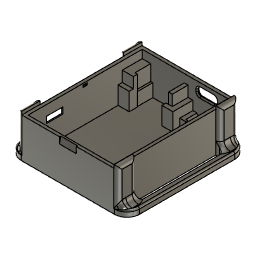
case 5.3 v6 (Autodesk Fusion 360 design; units mm, degrees)
Autodesk Fusion 360 part; units mm, degrees
note: some values were not read from the file. Set by a fixed rule: which face or edge a step refers to.
sketch "case" plane through (0, 0, 0) normal (0, 0, 1) x (1, 0, 0) in component "case"
  line L0 (0, 0) -> (41, 0)
  line L1 (41, 0) -> (41, 41)
  line L2 (0, 41) -> (0, 0)
  line L3 (0, 41) -> (0, 54.6)
  line L4 (0, 54.6) -> (41, 54.6)
  line L5 (41, 54.6) -> (41, 41)
  line L6 (4.1, 47.05) -> (0, 47.05)
  line L7 (4.1, 47.05) -> (4.1, 54.6)
  line L8 (20.15, 47.05) -> (4.1, 47.05)
  line L9 (20.15, 54.6) -> (20.15, 47.05)
  line L10 (0, 45.05) -> (5.3, 45.05)
  line L11 (5.3, 45.05) -> (5.3, 47.05)
  line L12 (12.125, 47.05) -> (12.125, 54.6) construction
  line L13 (24.25, 45.05) -> (18.95, 45.05)
  line L14 (18.95, 45.05) -> (18.95, 47.05)
  line L15 (20.15, 47.05) -> (24.25, 47.05)
  line L16 (24.25, 45.05) -> (24.25, 54.6)
  line L17 (41, 41) -> (0.0428, 41) construction
  line L18 (39, 43) -> (39, 54.6)
  line L19 (41, 41) -> (36, 41)
  line L20 (36, 41) -> (36, 43)
  line L21 (36, 43) -> (39, 43)
  line L22 (5.1, 47.05) -> (5.1, 54.6)
  line L23 (19.15, 47.05) -> (19.15, 54.6)
  line L24 (36, 43) -> (36, 45)
  line L25 (36, 45) -> (39, 45)
  line L26 (39, 43) -> (41, 43)
  line L27 (0, 2) -> (41, 2)
  line L28 (0, 43.05) -> (5.3, 43.05)
  line L29 (5.3, 45.05) -> (5.3, 43.05)
  dimension "d1" = 41
  dimension "d2" = 41
  dimension "d268" = 16.05
  dimension "d269" = 7.55
  dimension "d270" = 13.6
  dimension "d274" = 2
  dimension "d275" = 1.2
  dimension "d329" = 2
  dimension "d330" = 2
  dimension "d336" = 4.1
  dimension "d338" = 1
  dimension "d373" = 2
  dimension "d374" = 5
  dimension "d375" = 2
  dimension "d494" = 2
  constraint horizontal L0
  constraint vertical L1
  constraint vertical L2
  constraint coincident L0.start L2.end
  constraint vertical L3
  constraint horizontal L4
  constraint vertical L5
  constraint vertical L9
  constraint horizontal L8
  constraint vertical L7
  constraint perpendicular L6 L7
  constraint coincident L3 L6.end
  constraint coincident L4 L7.end
  constraint coincident L4 L9.start
  constraint coincident L3 L10.start
  constraint perpendicular L3 L10
  constraint coincident L8 L11.end
  constraint perpendicular L8 L11
  constraint midpoint L8 L12.start
  constraint coincident L4 L12.end
  constraint perpendicular L4 L12
  constraint symmetric L6.start L12 L8.start
  constraint symmetric L6.end L12 L15.end
  constraint symmetric L10.start L12 L13.start
  constraint symmetric L10.end L12 L13.end
  constraint symmetric L11.end L12 L14.end
  constraint coincident L4 L16.end
  constraint perpendicular L4 L16
  constraint perpendicular L5 L17
  constraint collinear L1.end L2.start L17.end
  constraint coincident L4 L18.end
  constraint perpendicular L4 L18
  constraint coincident L17 L19.end
  constraint perpendicular L17 L20
  constraint perpendicular L20 L21
  constraint coincident L18.start L21
  constraint coincident L8 L22.start
  constraint coincident L4 L22.end
  constraint perpendicular L4 L22
  constraint symmetric L12 L22.start L23.start
  constraint symmetric L12 L22.end L23.end
  constraint perpendicular L21 L24
  constraint coincident L18 L25.end
  constraint perpendicular L18 L25
  constraint coincident L5 L26.end
  constraint parallel L21 L26
  constraint coincident L2 L27.start
  constraint coincident L1 L27.end
  constraint perpendicular L1 L27
  constraint coincident L3 L28.start
  constraint perpendicular L3 L28
  constraint perpendicular L28 L29
  measures "d1" distance of L0.start L0.end
  measures "d2" distance of L0.start L2.start
  measures "d268" distance of L7.end L9.start
  measures "d269" distance of L6.start L7.end
  measures "d270" distance of L2.start L4
  measures "d274" distance of L6 L10
  measures "d275" distance of L7 L11
  measures "d329" distance of L5 L18
  measures "d330" distance of L19 L21
  measures "d336" distance of L3 L7
  measures "d338" distance of L7 L22
  measures "d373" distance of L21 L25
  measures "d374" distance of L5 L24
  measures "d375" distance of L0 L27
  measures "d494" distance of L10 L28
extrude "Extrude1" add sketch "case" along normal blind 17.5 makes body 1 in component "case"
shell "Shell1" thickness 1.5 outward yes removed faces 1 at (13.6667, 28, 17.5) on bodies 1 in component "case"
extrude "Extrude21" add sketch "case" along normal blind 8.5 contours L0 L1 L2 L27 | L3 L10 L28 L29 | L4 L5 L18 L26 | L18 L21 L24 L25 | L4 L9 L15 L16 | L8 L13 L14 L15 L16 bodies 1 in component "case"
extrude "Extrude22" add sketch "case" along normal blind 13.6 contours L3 L6 L8 L10 L11 | L3 L4 L6 L7 bodies 1 in component "case"
extrude "Extrude25" add sketch "case" along normal blind 6.2 contours L4 L7 L8 L22 | L4 L8 L9 L23 bodies 1 in component "case"
sketch "tray" plane through (0, 0, 0) normal (0, 0, 1) x (1, 0, 0) in component "tray"
  line L0 (0, 0) -> (40.75, 0)
  line L1 (40.75, 0) -> (40.75, 54.3)
  line L2 (0, 54.3) -> (0, 0)
  line L3 (25.45, 25.8) -> (25.45, 27.6)
  line L4 (25.45, 27.6) -> (36.25, 27.6)
  line L5 (36.25, 27.6) -> (36.25, 25.8)
  line L6 (36.25, 25.8) -> (25.45, 27.6) construction
  line L7 (25.45, 25.8) -> (36.25, 27.6) construction
  line L8 (0, 43.7) -> (0, 27.5) construction
  line L9 (0, 54.3) -> (0, 43.7)
  line L10 (40.75, 54.3) -> (0, 54.3)
  line L11 (0, 25.8) -> (40.75, 25.8)
  line L12 (0, 12.9) -> (40.75, 12.9) construction
  line L13 (27.2, 6.65) -> (11.5, 6.65)
  line L14 (11.5, 6.65) -> (11.5, 19.15)
  line L15 (11.5, 19.15) -> (27.2, 19.15)
  line L16 (27.2, 19.15) -> (27.2, 6.65)
  line L17 (27.2, 6.65) -> (11.5, 19.15) construction
  line L18 (11.5, 6.65) -> (27.2, 19.15) construction
  line L19 (34.5, 4.7) -> (10, 4.7)
  line L20 (10, 4.7) -> (10, 21.1)
  line L21 (10, 21.1) -> (34.5, 21.1)
  line L22 (34.5, 21.1) -> (34.5, 4.7)
  line L23 (34.5, 4.7) -> (10, 21.1) construction
  line L24 (10, 4.7) -> (34.5, 21.1) construction
  line L25 (32.3, 25.8) -> (34.5, 23.6)
  line L26 (34.5, 21.1) -> (34.5, 25.8)
  line L27 (32.3, 0) -> (34.5, 2.2)
  line L28 (34.5, 4.7) -> (34.5, 0)
  line L29 (7.097, 0) -> (7.097, 3)
  line L30 (7.097, 3) -> (28.483, 3)
  line L31 (28.483, 3) -> (28.483, 0)
  line L32 (7.097, 0) -> (28.483, 0)
  line L33 (7.097, 25.8) -> (28.483, 25.8)
  line L34 (28.483, 22.8) -> (28.483, 25.8)
  line L35 (7.097, 22.8) -> (28.483, 22.8)
  line L36 (7.097, 25.8) -> (7.097, 22.8)
  line L37 (39.55, 25.8) -> (39.55, 54.3)
  line L38 (39.55, 40.05) -> (22.15, 40.05) construction
  line L39 (22.15, 25.8) -> (22.15, 54.3)
  line L40 (30.85, 40.05) -> (30.85, 25.8) construction
  line L41 (34.5, 23.6) -> (40.75, 23.6)
  line L42 (36.15, 54.3) -> (36.15, 50.9)
  line L43 (36.15, 50.9) -> (39.55, 50.9)
  line L44 (25.55, 50.9) -> (22.15, 50.9)
  line L45 (25.55, 54.3) -> (25.55, 50.9)
  line L46 (22.15, 27.9) -> (39.55, 27.9)
  line L47 (22.15, 31.3) -> (39.55, 31.3)
  line L48 (0, 25.8) -> (0, 0) construction
  line L49 (25.45, 25.8) -> (36.25, 25.8)
  line L50 (4.2, 54.3) -> (20.2, 54.3)
  line L51 (20.2, 54.3) -> (20.2, 46.5)
  line L52 (20.2, 46.5) -> (4.2, 46.5)
  line L53 (4.2, 46.5) -> (4.2, 54.3)
  line L54 (4.2, 46.5) -> (0, 46.5)
  line L55 (20.2, 46.5) -> (22.15, 46.5)
  line L56 (20.8, 46.5) -> (20.8, 25.8)
  line L57 (0, 42.9) -> (20.8, 42.9)
  line L58 (0, 27) -> (20.8, 27)
  line L59 (20.8, 39.9) -> (10, 39.9)
  line L60 (10, 39.9) -> (10, 42.9)
  line L61 (20.8, 46.5) -> (20.8, 54.3)
  line L62 (22.15, 50.9) -> (20.8, 50.9)
  line L63 (0, 44.1) -> (5.2, 44.1)
  line L64 (5.2, 44.1) -> (5.2, 42.9)
  line L65 (20.8, 27) -> (22.15, 27)
  line L66 (25.45, 27) -> (36.25, 27)
  line L67 (5.2, 44.1) -> (10, 44.1)
  line L68 (10, 42.9) -> (10, 44.1)
  circle A0 centre (18.1, 29.6) radius 1.4
  line L69 (0, 29.6) -> (20.8, 29.6) construction
  line L70 (10.4, 29.6) -> (10.4, 27)
  line L71 (20.8, 44.1) -> (18.8, 44.1)
  line L72 (18.8, 44.1) -> (18.8, 42.9)
  circle A1 centre (2.7, 29.6) radius 1.4
  line L73 (36.25, 25.8) -> (36.25, 23.6)
  line L74 (27.2, 19.15) -> (30.4, 19.15)
  line L75 (30.4, 19.15) -> (30.4, 6.65)
  line L76 (30.4, 6.65) -> (27.2, 6.65)
  line L77 (28.483, 3) -> (28.483, 22.8)
  point P0 (30.85, 26.7)
  point P1 (19.35, 12.9)
  point P2 (22.25, 12.9)
  point P3 (61.6964, 12.9)
  point P4 (8.897, 1.47)
  point P5 (26.683, 1.47)
  dimension "d38" = 40.75
  dimension "d46" = 10.8
  dimension "d141" = 12.5
  dimension "d142" = 11.5
  dimension "d143" = 27.2
  dimension "d144" = 10
  dimension "d145" = 34.5
  dimension "d146" = 16.4
  dimension "d199" = 54.3
  dimension "d212" = 8.897
  dimension "d213" = 17.786
  dimension "d214" = 1.47
  dimension "d215" = 1.8
  dimension "d216" = 1.8
  dimension "d217" = 3
  dimension "d218" = 1.47
  dimension "d222" = 17.4
  dimension "d224" = 25.8
  dimension "d226" = 3.4
  dimension "d227" = 3.4
  dimension "d229" = 23
  dimension "d244" = 26.4
  dimension "d246" = 26.7
  dimension "d247" = 45
  dimension "d248" = 1.8
  dimension "d249" = 32.3
  dimension "d253" = 1.2
  dimension "d254" = 16
  dimension "d255" = 7.8
  dimension "d256" = 4.2
  dimension "d257" = 9.9
  dimension "d259" = 20.8
  dimension "d261" = 1.2
  dimension "d262" = 15.9
  dimension "d263" = 10.8
  dimension "d264" = 3
  dimension "d265" = 5.2
  dimension "d266" = 1.2
  dimension "d323" = 2.8
  dimension "d326" = 2.6
  dimension "d353" = 2.7
  dimension "d354" = 2
  dimension "d363" = 28.5
  dimension "d364" = 2.2
  dimension "d365" = 24.5
  dimension "d366" = 1.5
  dimension "d367" = 15.7
  dimension "d459" = 3.2
  constraint horizontal L0
  constraint vertical L1
  constraint horizontal L10
  constraint collinear L0.start L2.end L0.end
  constraint coincident L6 P0
  constraint coincident L7 P0
  constraint coincident L2 L8.end
  constraint vertical L9
  constraint coincident L2 L12.start
  constraint coincident L1 L12.end
  constraint perpendicular L1 L12
  constraint horizontal L13
  constraint perpendicular L13 L14
  constraint parallel L13 L15
  constraint parallel L14 L16
  constraint coincident L17 P1
  constraint coincident L18 P1
  constraint coincident L12 P1
  constraint horizontal L19
  constraint perpendicular L19 L20
  constraint parallel L19 L21
  constraint parallel L20 L22
  constraint coincident L23 P2
  constraint coincident L24 P2
  constraint coincident L12 P2
  constraint perpendicular L21 L26
  constraint coincident L25.end L26
  constraint symmetric L12 L21.end L19.start
  constraint symmetric L12 L25.start L27.start
  constraint symmetric L12 L25.end L27.end
  constraint symmetric L12 L26.end L28.end
  constraint coincident L12 P3
  constraint coincident L0 L29.start
  constraint perpendicular L0 L29
  constraint perpendicular L29 L30
  constraint coincident L0 L31.end
  constraint perpendicular L0 L31
  constraint symmetric L12 L29.start L33.start
  constraint symmetric L12 L29.end L35.start
  constraint symmetric L12 L30.end L34.start
  constraint symmetric L12 L31.end L33.end
  constraint coincident L10 L37.end
  constraint perpendicular L10 L37
  constraint coincident L2.start L10
  constraint midpoint L37 L38.start
  constraint perpendicular L37 L38
  constraint coincident L11 L39.start
  constraint coincident L10 L39.end
  constraint perpendicular L10 L39
  constraint coincident L38.end L39
  constraint vertical L40
  constraint midpoint L38 L40.start
  constraint coincident P0 L40
  constraint coincident L1 L41.end
  constraint perpendicular L1 L41
  constraint coincident L10 L42.start
  constraint perpendicular L10 L42
  constraint coincident L37 L43.end
  constraint perpendicular L37 L43
  constraint symmetric L40 L42.start L45.start
  constraint symmetric L40 L42.end L44.start
  constraint symmetric L40 L43.end L44.end
  constraint coincident L39 L46.start
  constraint coincident L37 L46.end
  constraint perpendicular L37 L46
  constraint coincident L39 L47.start
  constraint coincident L37 L47.end
  constraint perpendicular L39 L47
  constraint midpoint L12.start L48
  constraint coincident L1 L11.end
  constraint midpoint L7 P0
  constraint perpendicular L5 L49
  constraint coincident L11 L25.start
  constraint horizontal L50
  constraint vertical L51
  constraint horizontal L52
  constraint vertical L53
  constraint coincident L10 L50.start
  constraint coincident L9 L54.end
  constraint perpendicular L53 L54
  constraint coincident L39 L55.end
  constraint perpendicular L39 L55
  constraint vertical L56
  constraint coincident L55 L56.start
  constraint coincident L11 L56.end
  constraint coincident L8 L57.start
  constraint coincident L56 L57.end
  constraint perpendicular L56 L57
  constraint coincident L2 L58.start
  constraint coincident L56 L58.end
  constraint perpendicular L56 L58
  constraint coincident L56 L59.start
  constraint perpendicular L56 L59
  constraint coincident L57 L60.end
  constraint perpendicular L57 L60
  constraint coincident L10 L61.end
  constraint perpendicular L10 L61
  constraint coincident L61 L62.end
  constraint perpendicular L61 L62
  constraint coincident L9 L63.start
  constraint perpendicular L9 L63
  constraint coincident L57 L64.end
  constraint perpendicular L57 L64
  constraint collinear L11 L49
  constraint coincident L39 L65.end
  constraint perpendicular L39 L65
  constraint coincident L3 L66.start
  constraint coincident L5 L66.end
  constraint perpendicular L5 L66
  constraint collinear L65 L66
  constraint perpendicular L56 L67
  constraint perpendicular L57 L68
  constraint coincident L67.end L68
  constraint coincident L8 L69.start
  constraint coincident L56 L69.end
  constraint perpendicular L56 L69
  constraint coincident A0.centre L69
  constraint midpoint L69 L70.start
  constraint midpoint L58 L70.end
  constraint coincident L56 L71.start
  constraint perpendicular L56 L71
  constraint coincident L57 L72.end
  constraint perpendicular L57 L72
  constraint collinear L67 L71
  constraint symmetric A0 L70 A1
  constraint coincident L41 L73.end
  constraint perpendicular L41 L73
  constraint perpendicular L16 L74
  constraint perpendicular L74 L75
  constraint perpendicular L16 L76
  constraint coincident L0.start L2.end
  measures "d38" distance of L0.start L0.end
  measures "d46" distance of L3 L5
  measures "d141" distance of L13.end L14.end
  measures "d142" distance of L2 L14
  measures "d143" distance of L2 L16
  measures "d144" distance of L2 L20
  measures "d145" distance of L2 L22
  measures "d146" distance of L19 L21
  measures "d199" distance of L0 L10
  measures "d212" distance of L2 P4
  measures "d213" distance of P4 P5
  measures "d214" distance of L0 P4
  measures "d215" distance of P4 L29
  measures "d216" distance of P5 L31
  measures "d217" distance of L0 L30
  measures "d218" distance of L0 P5
  measures "d222" distance of L38.start L38.end
  measures "d224" distance of L0 L11
  measures "d226" distance of L42.end L43.end
  measures "d227" distance of L42.start L42.end
  measures "d229" distance of L10 L47
  measures "d244" distance of L10 L46
  measures "d246" distance of L4 L10
  measures "d247" angle of L11 L25
  measures "d248" distance of L4 L11
  measures "d249" distance of L2 L25.start
  measures "d253" distance of L1 L37
  measures "d254" distance of L50.start L50.end
  measures "d255" distance of L50.start L52.end
  measures "d256" distance of L2 L53
  measures "d257" distance of L1 L40
  measures "d259" distance of L2 L56
  measures "d261" distance of L11 L58
  measures "d262" distance of L57 L58
  measures "d263" distance of L59.start L59.end
  measures "d264" distance of L59.end L60.end
  measures "d265" distance of L63.start L63.end
  measures "d266" distance of L63.end L64.end
  measures "d323" diameter of A0
  measures "d326" distance of L58 L69
  measures "d353" distance of L56 A0.centre
  measures "d354" distance of L56 L72
  measures "d363" distance of L10 L33
  measures "d364" distance of L25.end L26.end
  measures "d365" distance of L20 L22
  measures "d366" distance of L14 L20
  measures "d367" distance of L14 L16
  measures "d459" distance of L15.end L74.end
extrude "Extrude6" add sketch "tray" against normal blind 1.55 separate body contours L0 L2 L11 L19 L20 L21 L29 L30 L35 L36 L77 | L2 L11 L33 L56 L58 | L0 L19 L27 L28 L31 L77 | L2 L56 L57 L58 L59 L60 | L0 L27 L28 | L2 L9 L57 L63 L64 | L11 L33 L39 L56 L65 | L19 L21 L22 L74 L75 L76 L77 | L13 L14 L15 L19 L20 L21 L74 L76 L77 | L39 L55 L56 L65 | L3 L4 L5 L11 L33 L37 L39 L46 | L11 L21 L25 L26 L34 L49 L77 | L74 L75 L76 L77 | L16 L74 L76 L77 | L3 L5 L11 L33 L49 L66 | L1 L11 L41 L73 | L13 L14 L15 L16 | L56 L57 L71 L72 | L3 L4 L5 L66 | L11 L25 L26 L49 | L1 L10 L11 L37 | L11 L26 L41 L49 L73 | L10 L37 L39 L42 L43 L44 L45 L47 | A0 | A1 makes body 2 in component "tray"
extrude "Extrude7" add sketch "tray" along normal blind 2.4 contours L2 L9 L57 L63 L64 | L39 L55 L56 L65 | L1 L11 L41 L73 | L56 L57 L71 L72 | L3 L4 L5 L66 | L1 L10 L11 L37 | L11 L26 L41 L49 L73 bodies 2 in component "tray"
extrude "Extrude1'" add sketch "tray" along normal blind 4 contours L2 L11 L33 L56 L58 | L0 L27 L28 | L11 L33 L39 L56 L65 | L3 L5 L11 L33 L49 L66 | L11 L25 L26 L49 | L11 L26 L41 L49 L73 bodies 2 in component "tray"
extrude "Extrude15" cut sketch "tray" along normal through all from surface at -0.55 contours L0 L2 L11 L19 L20 L21 L29 L30 L35 L36 L77 | L0 L19 L27 L28 L31 L77 | L19 L21 L22 L74 L75 L76 L77 | L13 L14 L15 L19 L20 L21 L74 L76 L77 | L11 L21 L25 L26 L34 L49 L77 | L74 L75 L76 L77 | L16 L74 L76 L77 | L13 L14 L15 L16 bodies 2 in component "tray"
sketch "switch shoulder" plane through (0, 0, 8.5) normal (0, 0, 1) x (-1, 0, 0) in component "case"
  line L0 (-18.95, -45.05) -> (-24.25, -45.05)
  line L1 (-24.25, -45.05) -> (-24.25, -54.6)
  line L2 (-24.25, -54.6) -> (-20.15, -54.6)
  line L3 (-20.15, -54.6) -> (-20.15, -47.05)
  line L4 (-20.15, -47.05) -> (-18.95, -47.05)
  line L5 (-18.95, -47.05) -> (-18.95, -45.05)
  line L6 (-22.25, -51.05) -> (-25.65, -51.05)
  line L7 (-22.25, -46.65) -> (-22.25, -51.05)
  line L8 (-20.9, -46.65) -> (-22.25, -46.65)
  line L9 (-20.15, -47.05) -> (-21.95, -47.05)
  line L10 (-21.95, -47.05) -> (-21.95, -54.6)
  line L11 (-20.9, -44.25) -> (-20.9, -46.65)
  line L12 (-20.9, -40.05) -> (-20.9, -43.05)
  dimension "d304" = 1.8
  constraint coincident L3.end L4.start
  constraint perpendicular L3 L9
  constraint coincident L2 L10.end
  constraint perpendicular L2 L10
  measures "d304" distance of L3 L10
extrude "Extrude24" add sketch "switch shoulder" along normal up to surface (5.1 mm away) contours L2 L3 L9 L10 bodies 1 in component "case"
sketch "usb c" plane through (0, 54.6, 0) normal (0, -1, 0) x (1, 0, 0) in component "case"
  line L0 (0, 13.6) -> (4.1, 13.6)
  line L1 (4.1, 13.6) -> (4.1, 6.2)
  line L2 (5.1, 0) -> (19.15, 0)
  line L3 (20.15, 6.2) -> (20.15, 13.6)
  line L4 (21.95, 8.5) -> (24.25, 8.5)
  line L5 (24.25, 8.5) -> (24.25, 0)
  line L6 (24.25, 0) -> (39, 0)
  line L7 (41, 8.5) -> (41, 17.5)
  line L8 (41, 17.5) -> (0, 17.5)
  line L9 (0, 17.5) -> (0, 13.6)
  line L10 (34.2, 11.6) -> (27.6, 11.6)
  arc A0 (26.3, 12.9) -> (27.6, 11.6) centre (27.6, 12.9) ccw
  line L11 (26.3, 12.9) -> (26.3, 13.9)
  arc A1 (27.6, 15.2) -> (26.3, 13.9) centre (27.6, 13.9) ccw
  line L12 (27.6, 15.2) -> (34.2, 15.2)
  arc A2 (35.5, 13.9) -> (34.2, 15.2) centre (34.2, 13.9) ccw
  line L13 (35.5, 13.9) -> (35.5, 12.9)
  arc A3 (34.2, 11.6) -> (35.5, 12.9) centre (34.2, 12.9) ccw
  line L14 (26.3, 13.4) -> (35.5, 13.4) construction
  line L15 (24.25, 8.5) -> (41, 8.5) construction
  line L16 (30.9, 13.4) -> (30.9, 8.5) construction
  line L17 (39, 0) -> (39, 8.5)
  line L18 (39, 8.5) -> (41, 8.5)
  line L19 (5.1, 6.2) -> (5.1, 0)
  line L20 (19.15, 0) -> (19.15, 6.2)
  line L21 (19.15, 6.2) -> (20.15, 6.2)
  line L22 (4.1, 6.2) -> (5.1, 6.2)
  line L23 (30.9, 8.5) -> (30.9, 0) construction
  line L24 (21.95, 13.6) -> (21.95, 8.5)
  line L25 (20.15, 13.6) -> (21.95, 13.6)
  point P0 (30.9, 13.4)
  point P1 (30.9, 10.1)
  dimension "d280" = 9.2
  dimension "d281" = 3.6
  dimension "d282" = 1.3
  dimension "d283" = 10.1
  dimension "d288" = 1.6
  dimension "d289" = 1.5
  constraint horizontal L10
  constraint vertical L11
  constraint horizontal L12
  constraint vertical L13
  constraint tangent L12 A2
  constraint tangent A2 L13
  constraint tangent L13 A3
  constraint tangent L10 A3
  constraint equal A2 A3
  constraint tangent L10 A0
  constraint tangent A0 L11
  constraint equal A0 A2
  constraint tangent L11 A1
  constraint tangent A1 L12
  constraint equal A1 A2
  constraint midpoint L14.start L11
  constraint midpoint L14.end L13
  constraint midpoint L14 P0
  constraint coincident L4.end L5.start
  constraint coincident L7 L15.end
  constraint perpendicular L7 L15
  constraint coincident P0 L16.start
  constraint coincident L15 L16.end
  constraint perpendicular L15 L16
  constraint coincident L16 P1
  constraint coincident L6 L23.end
  constraint perpendicular L6 L23
  measures "d280" distance of L11 L13
  measures "d281" distance of L10 L12
  measures "d282" radius of A2
  measures "d283" distance of L7 P0
  measures "d288" distance of L15 P1
  measures "d289" distance of L10 P1
extrude "Extrude23" cut sketch "usb c" against normal through all contours L10 A0 L11 A1 L12 A2 L13 A3 bodies 1 in component "case"
chamfer "Chamfer3" distance 0.6 angle 45 16 edges at (30.9, 54.6, 15.2) (35.1192, 54.6, 14.8192) (35.5, 54.6, 13.4) (35.1192, 54.6, 11.9808) (30.9, 54.6, 11.6) (26.6808, 54.6, 11.9808) (26.3, 54.6, 13.4) (26.6808, 54.6, 14.8192) (30.9, 56.1, 15.2) (26.6808, 56.1, 14.8192) (26.3, 56.1, 13.4) (26.6808, 56.1, 11.9808) (30.9, 56.1, 11.6) (35.1192, 56.1, 11.9808) (35.5, 56.1, 13.4) (35.1192, 56.1, 14.8192) on bodies 1 in component "case"
sketch "lid" plane through (0, 0, 0) normal (0, 0, 1) x (1, 0, 0) in component "lid"
  line L0 (41, 54.6) -> (0, 54.6)
  line L1 (41, 54.6) -> (41, 0)
  line L2 (41, 0) -> (0, 0)
  line L3 (0, 0) -> (0, 54.6)
  line L4 (42.5, 56.1) -> (-1.5, 56.1)
  line L5 (-1.5, -1.5) -> (-1.5, 56.1)
  line L6 (42.5, -1.5) -> (-1.5, -1.5)
  line L7 (42.5, 56.1) -> (42.5, -1.5)
  line L8 (1.25, 1.25) -> (1.25, 53.35)
  line L9 (39.75, 53.35) -> (1.25, 53.35)
  line L10 (39.75, 53.35) -> (39.75, 1.25)
  line L11 (39.75, 1.25) -> (1.25, 1.25)
  line L12 (20.15, 54.6) -> (20.15, 47.05) construction
  line L13 (4.1, 47.05) -> (4.1, 54.6) construction
  line L14 (4.1, 54.6) -> (20.15, 54.6) construction
  line L15 (4.1, 47.05) -> (20.15, 47.05) construction
  line L16 (12.125, 47.05) -> (12.125, 54.6) construction
  line L17 (16.725, 48.725) -> (7.525, 48.725)
  line L18 (7.525, 48.725) -> (7.525, 52.925)
  line L19 (7.525, 52.925) -> (16.725, 52.925)
  line L20 (16.725, 52.925) -> (16.725, 48.725)
  line L21 (16.725, 48.725) -> (7.525, 52.925) construction
  line L22 (7.525, 48.725) -> (16.725, 52.925) construction
  line L23 (0, 49.35) -> (1.25, 49.35)
  line L24 (20.5, 1.25) -> (20.5, 53.35) construction
  line L25 (1.25, 27.3) -> (39.75, 27.3) construction
  line L26 (0, 33.3) -> (1.25, 33.3)
  line L27 (0, 5.25) -> (1.25, 5.25)
  line L28 (0, 21.3) -> (1.25, 21.3)
  line L29 (41, 49.35) -> (39.75, 49.35)
  line L30 (41, 33.3) -> (39.75, 33.3)
  line L31 (41, 21.3) -> (39.75, 21.3)
  line L32 (41, 5.25) -> (39.75, 5.25)
  line L33 (0.25, 0.25) -> (0.25, 54.35)
  line L34 (40.75, 54.35) -> (0.25, 54.35)
  line L35 (40.75, 54.35) -> (40.75, 0.25)
  line L36 (40.75, 0.25) -> (0.25, 0.25)
  line L37 (37, 54.35) -> (37, 53.35)
  line L38 (24.8, 54.35) -> (24.8, 53.35)
  line L39 (6.925, 48.125) -> (17.325, 48.125)
  line L40 (6.925, 48.125) -> (6.925, 53.35)
  line L41 (17.325, 48.125) -> (17.325, 53.35)
  line L42 (6.175, 47.375) -> (6.175, 53.35)
  line L43 (6.175, 47.375) -> (18.075, 47.375)
  line L44 (18.075, 47.375) -> (18.075, 53.35)
  line L45 (1.25, 53.35) -> (0.25, 53.35)
  line L46 (39.75, 53.35) -> (40.75, 53.35)
  line L47 (39.75, 1.25) -> (40.75, 1.25)
  line L48 (1.25, 1.25) -> (0.25, 1.25)
  point P0 (12.125, 50.825)
  point P1 (35.5, 54.6)
  point P2 (26.3, 54.6)
  point P3 (12.125, 48.125)
  dimension "d310" = -1.5
  dimension "d311" = 1.25
  dimension "d318" = 9.2
  dimension "d319" = 4.2
  dimension "d332" = 4
  dimension "d333" = 6
  dimension "d362" = 0.25
  dimension "d368" = 1.5
  dimension "d369" = 1.5
  dimension "d370" = 0.6
  dimension "d371" = 0.6
  dimension "d372" = -0.75
  constraint coincident L13.end L14.start
  constraint coincident L12.start L14.end
  constraint coincident L13.start L15.start
  constraint coincident L12.end L15.end
  constraint midpoint L15 L16.start
  constraint midpoint L14 L16.end
  constraint horizontal L17
  constraint perpendicular L17 L18
  constraint parallel L17 L19
  constraint parallel L18 L20
  constraint coincident L21 P0
  constraint coincident L22 P0
  constraint midpoint L16 P0
  constraint coincident L3 L23.start
  constraint coincident L8 L23.end
  constraint perpendicular L8 L23
  constraint midpoint L11 L24.start
  constraint midpoint L9 L24.end
  constraint midpoint L8 L25.start
  constraint midpoint L10 L25.end
  constraint coincident L3 L26.start
  constraint coincident L8 L26.end
  constraint perpendicular L8 L26
  constraint symmetric L23.start L25 L27.start
  constraint symmetric L23.end L25 L27.end
  constraint symmetric L25 L26.start L28.start
  constraint symmetric L25 L26.end L28.end
  constraint symmetric L23.start L24 L29.start
  constraint symmetric L23.end L24 L29.end
  constraint symmetric L24 L26.start L30.start
  constraint symmetric L24 L26.end L30.end
  constraint symmetric L24 L27.start L32.start
  constraint symmetric L24 L27.end L32.end
  constraint symmetric L24 L28.start L31.start
  constraint symmetric L24 L28.end L31.end
  constraint coincident L34 L37.start
  constraint coincident L9 L37.end
  constraint perpendicular L9 L37
  constraint coincident L34 L38.start
  constraint coincident L9 L38.end
  constraint perpendicular L9 L38
  constraint perpendicular L16 L39
  constraint midpoint L39 P3
  constraint coincident L16 P3
  constraint coincident L9 L40.end
  constraint perpendicular L9 L40
  constraint coincident L9 L41.end
  constraint perpendicular L9 L41
  constraint coincident L33 L45.end
  constraint perpendicular L33 L45
  constraint coincident L35 L46.end
  constraint perpendicular L35 L46
  constraint coincident L35 L47.end
  constraint perpendicular L35 L47
  constraint coincident L33 L48.end
  constraint perpendicular L33 L48
  measures "d318" distance of L18.end L19.end
  measures "d319" distance of L17.end L18.end
  measures "d332" distance of L9 L23
  measures "d333" distance of L25 L26
  measures "d368" distance of P2 L38
  measures "d369" distance of P1 L37
  measures "d370" distance of L17 L39
  measures "d371" distance of L20 L41
extrude "Extrude1''" add sketch "lid" along normal blind 1.5 separate body contours L0 L1 L3 L23 L29 L33 L34 L35 | L1 L29 L30 L35 | L3 L23 L26 L33 | L1 L30 L31 L35 | L10 L29 L30 L35 | L10 L29 L35 L46 | L3 L26 L28 L33 | L8 L23 L33 L45 | L8 L23 L26 L33 | L1 L31 L32 L35 | L10 L30 L31 L35 | L8 L9 L10 L11 L42 L43 L44 | L9 L34 L35 L37 L46 | L3 L27 L28 L33 | L8 L26 L28 L33 | L9 L33 L34 L38 L45 | L1 L2 L3 L27 L32 L33 L35 L36 | L10 L31 L32 L35 | L8 L27 L28 L33 | L10 L32 L35 L47 | L9 L34 L37 L38 | L8 L27 L33 L48 | L9 L39 L40 L41 L42 L43 L44 | L11 L33 L35 L36 L47 L48 | L9 L39 L40 L41 | L4 L5 L6 L7 | L17 L18 L19 L20 makes body 3 in component "lid"
extrude "Extrude2" add sketch "lid" against normal blind 1.6 contours L9 L34 L35 L37 L46 | L9 L33 L34 L38 L45 | L9 L39 L40 L41 L42 L43 L44 | L11 L33 L35 L36 L47 L48 bodies 3 in component "lid"
extrude "Extrude4" add sketch "lid" against normal blind 2.4 contours L1 L30 L31 L35 | L3 L26 L28 L33 | L10 L30 L31 L35 | L8 L26 L28 L33 bodies 3 in component "lid"
extrude "Extrude3" cut sketch "lid" along normal through all contours L17 L18 L19 L20 bodies 3 in component "lid"
chamfer "Chamfer1" distance 1 distance2 1 4 edges at (7.525, 50.825, 1.5) (12.125, 52.925, 1.5) (12.125, 48.725, 1.5) (16.725, 50.825, 1.5) measured on face at (19.2417, 15.2417, 1.5) measured on face at (19.2417, 15.2417, 1.5) measured on face at (19.2417, 15.2417, 1.5) measured on face at (19.2417, 15.2417, 1.5) on bodies 3 in component "lid"
sketch "snap pins" plane through (0, 0, -17) normal (-1, 0, 0) x (0, -1, 0) in component "lid"
  line L0 (-21.3, 17) -> (-33.3, 17)
  line L1 (-33.3, 17) -> (-33.3, 14.6)
  line L2 (-33.3, 14.6) -> (-21.3, 14.6)
  line L3 (-21.3, 14.6) -> (-21.3, 17)
  line L4 (-33.3, 15.8) -> (-21.3, 15.8) construction
  line L5 (-26.5, 15.5) -> (-28.1, 15.5)
  line L6 (-28.1, 15.5) -> (-28.1, 16.1)
  line L7 (-28.1, 16.1) -> (-26.5, 16.1)
  line L8 (-26.5, 16.1) -> (-26.5, 15.5)
  line L9 (-26.5, 15.5) -> (-28.1, 16.1) construction
  line L10 (-28.1, 15.5) -> (-26.5, 16.1) construction
  line L11 (-27.3, 14.6) -> (-27.3, 17) construction
  point P0 (-27.3, 15.8)
  dimension "d341" = 0.6
  dimension "d342" = 1.6
  constraint midpoint L1 L4.start
  constraint midpoint L3 L4.end
  constraint horizontal L5
  constraint perpendicular L5 L6
  constraint parallel L5 L7
  constraint parallel L6 L8
  constraint coincident L9 P0
  constraint coincident L10 P0
  constraint coincident L4 P0
  constraint midpoint L2 L11.start
  constraint midpoint L0 L11.end
  constraint midpoint L4 P0
  measures "d341" distance of L5 L7
  measures "d342" distance of L6 L8
extrude "Extrude5" add sketch "snap pins" along normal blind 0.35 contours L5 L6 L7 L8 bodies 3 in component "lid"
ref_plane "WorkPlane1" through (20.5, 27.3, 0.75) normal (-1, 0, 0) x (0, -1, 0) in component "lid"
mirror "Mirror1" about plane through (20.5, 27.3, 0.75) normal (-1, 0, 0) of "Extrude5" in component "lid"
combine "Combine1" operation cut target body 1 tool bodies 3 body 3 seen with x (1, 0, 0) y (0, 1, 0) z (0, 0, 1) at (0, 0, 17.5) keep tools in component "case"
move_face "OffsetFaces2" offset -0.2 10 faces at (-0.2333, 27.5667, 16) (-0.1167, 26.5, 16.4) (-0.1167, 28.1, 16.2) (-0.2333, 27.0333, 16.6) (-0.35, 27.0333, 16.2) (41.35, 27.0333, 16.2) (41.2333, 26.5, 16.4) (41.1167, 27.0333, 16) (41.2333, 28.1, 16.2) (41.1167, 27.5667, 16.6) on bodies 1 in component "case"
fillet "Fillet2" radius 0.25 4 faces at (-0.35, 27.0333, -1.3) (-0.35, 27.0333, -1.3) (41.35, 27.0333, -1.3) (41.35, 27.0333, -1.3) on bodies 3 in component "lid"
sketch "jst zh 5pin" plane through (0, 0, 0) normal (0, 0, 1) x (1, 0, 0) in component "case"
  line L0 (27.6, 54.6) -> (34.2, 54.6)
  line L1 (30.9, 54.6) -> (30.9, 44.155) construction
  line L2 (35.4, 49.45) -> (26.4, 49.45)
  line L3 (26.4, 49.45) -> (26.4, 54.45)
  line L4 (26.4, 54.45) -> (35.4, 54.45)
  line L5 (35.4, 54.45) -> (35.4, 49.45)
  line L6 (35.4, 49.45) -> (26.4, 54.45) construction
  line L7 (26.4, 49.45) -> (35.4, 54.45) construction
  line L8 (35.55, 49.3) -> (26.25, 49.3)
  line L9 (26.25, 49.3) -> (26.25, 54.6)
  line L10 (26.25, 54.6) -> (35.55, 54.6)
  line L11 (35.55, 54.6) -> (35.55, 49.3)
  line L12 (34.75, 49.3) -> (34.75, 48.3)
  line L13 (39, 43) -> (39, 54.6)
  line L14 (24.25, 45.05) -> (24.25, 54.6)
  line L15 (34.75, 48.3) -> (39, 48.3)
  line L16 (27.05, 49.3) -> (27.05, 48.3)
  line L17 (27.05, 48.3) -> (24.25, 48.3)
  line L18 (0, 54.6) -> (41, 54.6)
  point P0 (30.9, 51.95)
  dimension "d376" = 9
  dimension "d377" = 5
  dimension "d378" = -0.15
  dimension "d379" = 1
  dimension "d380" = 0.8
  dimension "d381" = 0.8
  constraint midpoint L0 L1.start
  constraint perpendicular L0 L1
  constraint horizontal L2
  constraint perpendicular L2 L3
  constraint parallel L2 L4
  constraint parallel L3 L5
  constraint coincident L6 P0
  constraint coincident L7 P0
  constraint coincident L1 P0
  constraint collinear L0 L10
  constraint coincident L8 L12.start
  constraint perpendicular L8 L12
  constraint coincident L13 L15.end
  constraint perpendicular L13 L15
  constraint coincident L8 L16.start
  constraint perpendicular L8 L16
  constraint coincident L14 L17.end
  constraint perpendicular L14 L17
  constraint equal L12 L16
  measures "d376" distance of L3.end L4.end
  measures "d377" distance of L2.end L3.end
  measures "d379" distance of L8 L15
  measures "d380" distance of L11 L12
  measures "d381" distance of L9 L16
extrude "Extrude26" add sketch "jst zh 5pin" along normal blind 4.2 contours L8 L9 L14 L16 L17 L18 | L8 L11 L12 L13 L15 L18 bodies 1 in component "case"
sketch "jst zh 5pin hole" plane through (0, 56.1, 0) normal (0, 1, 0) x (-1, 0, 0) in component "case"
  line L0 (-42.5, -1.5) -> (1.5, -1.5)
  line L1 (1.5, -1.5) -> (1.5, 17.5)
  line L2 (1.5, 17.5) -> (-42.5, 17.5)
  line L3 (-42.5, 17.5) -> (-42.5, -1.5)
  line L4 (-34.2, 15.8) -> (-27.6, 15.8)
  arc A0 (-25.7, 13.9) -> (-27.6, 15.8) centre (-27.6, 13.9) ccw
  line L5 (-25.7, 13.9) -> (-25.7, 12.9)
  arc A1 (-27.6, 11) -> (-25.7, 12.9) centre (-27.6, 12.9) ccw
  line L6 (-27.6, 11) -> (-34.2, 11)
  arc A2 (-36.1, 12.9) -> (-34.2, 11) centre (-34.2, 12.9) ccw
  line L7 (-36.1, 12.9) -> (-36.1, 13.9)
  arc A3 (-34.2, 15.8) -> (-36.1, 13.9) centre (-34.2, 13.9) ccw
  line L8 (-26.25, 0) -> (-35.55, 0)
  line L9 (-35.55, 0) -> (-35.55, 4.2)
  line L10 (-35.55, 4.2) -> (-39, 4.2)
  line L11 (-24.25, 4.2) -> (-26.25, 4.2)
  line L12 (-26.25, 4.2) -> (-26.25, 0)
  line L13 (-35.55, 4.2) -> (-26.25, 4.2)
  line L14 (-30.9, 0) -> (-30.9, 4.2) construction
  line L15 (-35.55, 3.6) -> (-26.25, 3.6)
  line L16 (-29.7, 5.2) -> (-32.1, 5.2)
  line L17 (-32.1, 5.2) -> (-32.1, 4.2)
  line L18 (-32.1, 4.2) -> (-29.7, 4.2)
  line L19 (-29.7, 4.2) -> (-29.7, 5.2)
  line L20 (-29.7, 5.2) -> (-32.1, 4.2) construction
  line L21 (-32.1, 5.2) -> (-29.7, 4.2) construction
  line L22 (-35.55, 0.6) -> (-26.25, 0.6)
  point P0 (-30.9, 4.7)
  dimension "d394" = 2.4
  dimension "d395" = 1
  dimension "d490" = 0.6
  dimension "d491" = 0.6
  constraint coincident L9.end L10.start
  constraint coincident L11.end L12.start
  constraint midpoint L8 L14.start
  constraint midpoint L13 L14.end
  constraint coincident L9 L15.start
  constraint horizontal L16
  constraint perpendicular L16 L17
  constraint parallel L16 L18
  constraint parallel L17 L19
  constraint coincident L20 P0
  constraint coincident L21 P0
  constraint collinear L13 L18
  constraint collinear L14.start L14.end P0
  constraint coincident L12 L15.end
  constraint coincident L9 L22.start
  constraint coincident L12 L22.end
  constraint perpendicular L12 L22
  measures "d394" distance of L17.end L18.end
  measures "d395" distance of L16.end L17.end
  measures "d490" distance of L13 L15
  measures "d491" distance of L8 L22
extrude "Extrude27" cut sketch "jst zh 5pin hole" against normal up to surface (1.5 mm away) contours L9 L12 L15 L22 bodies 1 in component "case"
extrude "Extrude28" cut sketch "jst zh 5pin hole" against normal up to surface (0.9 mm away) contours L8 L9 L12 L22 | L9 L12 L15 L22 | L9 L12 L13 L15 L18 bodies 1 in component "case"
chamfer "Chamfer4" distance 0.6 distance2 0.6 4 edges at (30.9, 56.1, 4.2) (26.25, 56.1, 2.1) (30.9, 56.1, 0) (35.55, 56.1, 2.1) measured on face at (7.5923, 56.1, 9.4549) measured on face at (7.5923, 56.1, 9.4549) measured on face at (7.5923, 56.1, 9.4549) measured on face at (7.5923, 56.1, 9.4549) on bodies 1 in component "case"
extrude "Extrude29" add sketch "jst zh 5pin hole" against normal blind 0.6 from surface at -1.5 contours L13 L16 L17 L18 L19 bodies 1 in component "case"
chamfer "Chamfer5" distance 1 distance2 0.6 1 edges at (30.9, 54, 5.2) measured on face at (31.3, 54, 4.8667) on bodies 1 in component "case"
ref_plane "WorkPlane2" through (20.5, 27.3, 8) normal (0, -1, 0) x (1, 0, 0) in component "case"
ref_plane "WorkPlane4" through (20.5, 27.3, 8) normal (1, 0, 0) x (0, 1, 0) in component "case"
sketch "buckle base" plane through (0, 0, -1.5) normal (0, 0, -1) x (1, 0, 0) in component "case"
  line L0 (-1.5, 1.5) -> (-1.5, -56.1)
  line L1 (-1.5, -56.1) -> (42.5, -56.1)
  line L2 (42.5, -56.1) -> (42.5, 1.5)
  line L3 (42.5, 1.5) -> (-1.5, 1.5)
  line L4 (42.5, -27.3) -> (48.8, -27.3) construction
  line L5 (46.3, -27.3) -> (46.3, -45.3)
  line L6 (48.8, -27.3) -> (48.8, -50.1)
  line L7 (44.3, -47.3) -> (42.5, -47.3)
  arc A0 (44.3, -47.3) -> (46.3, -45.3) centre (44.3, -45.3) ccw
  line L8 (42.8, -56.1) -> (42.5, -56.1)
  arc A1 (42.8, -56.1) -> (48.8, -50.1) centre (42.8, -50.1) ccw
  line L9 (42.5, -47.3) -> (42.5, -47.3)
  line L10 (44.5, -49.3) -> (44.5, -54.1)
  line L11 (42.5, -56.1) -> (42.5, -47.3)
  line L12 (42.5, -56.1) -> (42.5, -56.1)
  arc A2 (42.5, -56.1) -> (44.5, -54.1) centre (42.5, -54.1) ccw
  arc A3 (44.5, -49.3) -> (42.5, -47.3) centre (42.5, -49.3) ccw
  line L13 (46.3, -27.3) -> (48.8, -27.3)
  arc A4 (44.5, -0.5) -> (42.5, 1.5) centre (42.5, -0.5) ccw
  line L14 (44.3, -7.3) -> (42.5, -7.3)
  arc A5 (46.3, -9.3) -> (44.3, -7.3) centre (44.3, -9.3) ccw
  arc A6 (42.5, -7.3) -> (44.5, -5.3) centre (42.5, -5.3) ccw
  line L15 (42.8, 1.5) -> (42.5, 1.5)
  line L16 (44.5, -5.3) -> (44.5, -0.5)
  arc A7 (48.8, -4.5) -> (42.8, 1.5) centre (42.8, -4.5) ccw
  line L17 (46.3, -27.3) -> (46.3, -9.3)
  line L18 (46.3, -27.3) -> (48.8, -27.3)
  line L19 (48.8, -27.3) -> (48.8, -4.5)
  point P0 (44.5, -47.3)
  point P1 (44.5, -7.3)
  point P2 (42.5, 1.5)
  point P3 (42.5, -27.3)
  point P4 (42.5, 1.5)
  dimension "d416" = 3.8
  dimension "d417" = 2.5
  dimension "d473" = 2
  dimension "d474" = 20
  dimension "d475" = 6
  dimension "d476" = 2
  dimension "d477" = 2
  constraint midpoint L2 P3
  constraint perpendicular L2 L4
  constraint coincident L4 L5.start
  constraint perpendicular L4 L5
  constraint perpendicular L4 L6
  constraint coincident L2 L7.end
  constraint perpendicular L2 L7
  constraint tangent L5 A0
  constraint tangent L7 A0
  constraint coincident L1.end L2.start
  constraint perpendicular L2 L8
  constraint tangent L6 A1
  constraint tangent L8 A1
  constraint vertical L10
  constraint vertical L11
  constraint tangent L10 A2
  constraint coincident P0 L10
  constraint coincident P0 L9
  constraint tangent L10 A3
  constraint equal A2 A3
  constraint symmetric L1.end L4 P4
  constraint symmetric P3 L4 L4.start
  constraint symmetric L6.start L4 L13.end
  constraint symmetric L4 L5.start L13.start
  constraint symmetric L4 L7.end L14.end
  constraint symmetric L4 L5.end A5.start
  constraint symmetric L4 L7.start L14.start
  constraint symmetric L4 A0 A5
  constraint symmetric L4 L1.end P4
  constraint symmetric L4 L6.end A7.start
  constraint symmetric L4 L8.start L15.start
  constraint symmetric L4 A1 A7
  constraint symmetric L4 P0 P1
  constraint symmetric L4 L10.end A4.start
  constraint symmetric L4 A2 A4
  constraint symmetric L4 L10.start A6.end
  constraint symmetric L4 A3 A6
  measures "d416" distance of L2 L5
  measures "d417" distance of L5 L6
  measures "d473" radius of A0
  measures "d474" distance of L4 L7
  measures "d475" radius of A1
  measures "d476" distance of L7.end P0
  measures "d477" radius of A2
extrude "Extrude31" add sketch "buckle base" against normal up to surface (20.5 mm away) contours L2 A4 A6 L16 | L2 L10 L11 A2 A3 bodies 1 in component "case"
extrude "Extrude37" add sketch "buckle base" against normal blind 3 contours L13 A4 L14 A5 A6 L15 L16 A7 L17 L18 L19 | L5 L6 L7 A0 L8 A1 L10 A2 A3 L13 L18 bodies 1 in component "case"
fillet "Fillet10" radius 0.8 5 edges at (42.65, -1.5, 1.5) (47.0426, 0.2574, 1.5) (48.8, 27.3, 1.5) (47.0426, 54.3426, 1.5) (42.65, 56.1, 1.5) on bodies 1 in component "case"
fillet "Fillet11" radius 3 10 edges at (43.9142, 47.8858, 1.5) (44.5, 51.7, 1.5) (44.432, 54.6169, 1.5) (43.5832, 55.7812, 1.2949) (42.649, 56.0943, 0.7942) (42.649, -1.4943, 0.7942) (43.5603, -1.1958, 1.2845) (44.432, -0.0169, 1.5) (44.5, 2.9, 1.5) (43.9142, 6.7142, 1.5) on bodies 1 in component "case"
sketch "pillar chamfer" plane through (0, 56.1, 0) normal (0, 1, 0) x (-1, 0, 0) in component "case"
  line L0 (-42.8, -1.5) -> (1.5, -1.5)
  line L1 (1.5, -1.5) -> (1.5, 17.5)
  line L2 (-42.5, 17.5) -> (-42.5, 19)
  line L3 (-44.5, 19.8243) -> (-42.5, 19.8243)
  line L4 (-42.5, 19.8243) -> (-42.5, 19)
  line L5 (-42.5, 17.5) -> (-42.6, 17.5)
  line L6 (-42.6, 17.5) -> (-42.6, 19)
  line L7 (-44.5, 19.8243) -> (-44.5, 15.6793)
  line L8 (-44.5, 15.6793) -> (-42.5, 15.6793) construction
  line L9 (-42.6, 17.5) -> (-42.6, 15.6793) construction
  line L10 (-44.5, 17) -> (-42.6, 17)
  arc A0 (-42.6, 19) -> (-44.5, 17) centre (-42.4974, 17) ccw
  line L11 (-42.5, 17.5) -> (-42.5, 0.7)
  line L12 (-42.8, 0.7) -> (-42.8, -1.5)
  line L13 (1.5, 17.5) -> (-42.5, 17.5)
  line L14 (-34.2, 15.8) -> (-27.6, 15.8)
  arc A1 (-25.7, 13.9) -> (-27.6, 15.8) centre (-27.6, 13.9) ccw
  line L15 (-25.7, 13.9) -> (-25.7, 12.9)
  arc A2 (-27.6, 11) -> (-25.7, 12.9) centre (-27.6, 12.9) ccw
  line L16 (-27.6, 11) -> (-34.2, 11)
  arc A3 (-36.1, 12.9) -> (-34.2, 11) centre (-34.2, 12.9) ccw
  line L17 (-36.1, 12.9) -> (-36.1, 13.9)
  arc A4 (-34.2, 15.8) -> (-36.1, 13.9) centre (-34.2, 13.9) ccw
  line L18 (-25.65, -0.6) -> (-36.15, -0.6)
  line L19 (-36.15, -0.6) -> (-36.15, 4.8)
  line L20 (-36.15, 4.8) -> (-25.65, 4.8)
  line L21 (-25.65, 4.8) -> (-25.65, -0.6)
  line L22 (-42.5, 0.7) -> (-42.8, 0.7)
  dimension "d458" = 0.1
  dimension "d469" = 2
  constraint perpendicular L2 L3
  constraint coincident L2.end L4.end
  constraint perpendicular L3 L7
  constraint coincident L8 L9.end
  constraint perpendicular L8 L9
  constraint coincident L7 L10.start
  constraint coincident L6 L10.end
  constraint perpendicular L6 L10
  constraint tangent L7 A0
  measures "d458" distance of L2.start L5.end
  measures "d469" distance of L3.start L3.end
extrude "Extrude33" cut sketch "pillar chamfer" against normal through all contours L2 L3 L4 L5 L6 L7 A0 bodies 1 in component "case"
split "Split1" by plane through (42.5, 0, 0) normal (1, 0, 0) bodies 1 makes body 4 at (47.9667, 21.3, -1.5) in component "case"
mirror "Mirror4" about plane through (20.5, 27.3, 8) normal (1, 0, 0) of bodies 4 makes body 5 in component "case"
combine "Combine2" operation add target body 1 tool bodies 4 5 in component "case"
sketch "usb micro" plane through (0, 0, 0) normal (1, 0, 0) x (0, 1, 0) in component "case"
  line L0 (26.3, 15.8) -> (26.3, 16.8)
  line L1 (26.3, 16.8) -> (28.3, 16.8)
  line L2 (28.3, 16.8) -> (28.3, 15.8)
  line L3 (28.3, 15.8) -> (26.3, 15.8)
  line L4 (54.6, 17.5) -> (0, 17.5)
  line L5 (0, 17.5) -> (0, 8.5)
  line L6 (0, 8.5) -> (2, 8.5)
  line L7 (2, 8.5) -> (2, 0)
  line L8 (2, 0) -> (45.05, 0)
  line L9 (45.05, 0) -> (45.05, 13.6)
  line L10 (45.05, 13.6) -> (54.6, 13.6)
  line L11 (54.6, 13.6) -> (54.6, 17.5)
  line L12 (25.95, 9.6) -> (25.95, 14.15)
  line L13 (0, 8.5) -> (0, 17.5)
  line L14 (12.7, 11.8) -> (12.7, 17.5) construction
  line L15 (16.6, 9.6) -> (8.8, 9.6)
  line L16 (8.8, 9.6) -> (8.8, 12.6)
  line L17 (8.8, 12.6) -> (16.6, 12.6)
  line L18 (16.6, 12.6) -> (16.6, 9.6)
  line L19 (16.6, 9.6) -> (8.8, 12.6) construction
  line L20 (8.8, 9.6) -> (16.6, 12.6) construction
  line L21 (18.05, 17.5) -> (8.05, 17.5)
  line L22 (7.7, 8.1) -> (17.7, 8.1)
  line L23 (0.15, 9.6) -> (25.95, 9.6)
  line L24 (0, 17.5) -> (54.6, 17.5)
  line L25 (0.15, 9.6) -> (0, 9.6)
  line L26 (12.7, 8.1) -> (12.7, 9.6) construction
  line L27 (7.7, 8.1) -> (7.7, 14.1)
  line L28 (7.7, 14.1) -> (17.7, 14.1)
  line L29 (17.7, 14.1) -> (17.7, 8.1)
  line L30 (26.3, 15.8) -> (26.3, 16.8)
  line L31 (26.3, 16.8) -> (28.3, 16.8)
  line L32 (28.3, 16.8) -> (28.3, 15.8)
  line L33 (28.3, 15.8) -> (26.3, 15.8)
  line L34 (54.6, 17.5) -> (0, 17.5)
  line L35 (0, 17.5) -> (0, 8.5)
  line L36 (0, 8.5) -> (2, 8.5)
  line L37 (2, 8.5) -> (2, 0)
  line L38 (2, 0) -> (43.05, 0)
  line L39 (45.05, 8.5) -> (45.05, 13.6)
  line L40 (45.05, 13.6) -> (54.6, 13.6)
  line L41 (54.6, 13.6) -> (54.6, 17.5)
  line L42 (43.05, 0) -> (43.05, 8.5)
  line L43 (43.05, 8.5) -> (45.05, 8.5)
  point P0 (12.7, 11.1)
  point P1 (12.7, 11.1)
  point P2 (12.7, 8.1)
  dimension "d450" = 7.8
  dimension "d451" = 3
  dimension "d454" = 10
  dimension "d457" = 3
  dimension "d464" = 6
  dimension "d465" = 12.7
  constraint coincident L4 L14.end
  constraint perpendicular L4 L14
  constraint horizontal L15
  constraint perpendicular L15 L16
  constraint parallel L15 L17
  constraint parallel L16 L18
  constraint coincident L19 P1
  constraint coincident L20 P1
  constraint coincident L14 P1
  constraint horizontal L21
  constraint parallel L21 L22
  constraint coincident L4 L21.start
  constraint coincident P1 P0
  constraint midpoint L22 P2
  constraint coincident L14 P2
  constraint coincident L23.start L25.start
  constraint coincident L13 L25.end
  constraint perpendicular L13 L25
  constraint coincident P2 L26.start
  constraint perpendicular L15 L26
  constraint perpendicular L22 L27
  constraint perpendicular L14 L28
  constraint perpendicular L22 L29
  constraint collinear L15 L23
  measures "d450" distance of L16.end L17.end
  measures "d451" distance of L15.end L16.end
  measures "d454" distance of L22.start L22.end
  measures "d457" distance of P1 L22
  measures "d464" distance of L22.start L27.end
  measures "d465" distance of L5 P1
extrude "Extrude34" cut sketch "usb micro" against normal through all contours L15 L16 L17 L18 L23 bodies 1 in component "case"
extrude "Extrude35" cut sketch "usb micro" against normal through all from surface at -0.6 contours L15 L22 L23 L27 L29 | L16 L17 L18 L23 L27 L28 L29 bodies 1 in component "case"
extrude "Extrude3'" add sketch "tray" along normal blind 2.4 from surface at -0.55 contours L0 L19 L27 L28 L31 L77 | L19 L21 L22 L74 L75 L76 L77 | L11 L21 L25 L26 L34 L49 L77 | L74 L75 L76 L77 bodies 2 in component "tray"
sketch "hole trench" plane through (0, 0, 8.5) normal (0, 0, 1) x (-1, 0, 0) in component "case"
  line L0 (0, 0) -> (-41, 0)
  line L1 (-41, 0) -> (-41, -2)
  line L2 (-41, -2) -> (0, -2)
  line L3 (0, -2) -> (0, 0)
  line L4 (-7.197, -3.15) -> (-7.197, -0.15)
  line L5 (-28.583, -25.95) -> (-28.583, -0.15)
  line L6 (-28.583, -3.15) -> (-7.197, -3.15)
  line L7 (-41, 0) -> (0, 0)
  line L8 (-28.583, -0.15) -> (-28.583, 0)
  line L9 (-7.197, -0.15) -> (-7.197, 0)
  constraint coincident L5.end L8.start
  constraint coincident L7 L8.end
  constraint perpendicular L7 L8
  constraint coincident L4.end L9.start
  constraint coincident L7 L9.end
  constraint perpendicular L7 L9
extrude "Extrude36" cut sketch "hole trench" against normal blind 1 contours L0 L2 L4 L5 L7 L8 L9 | L2 L4 L5 L6 bodies 1 in component "case"
sketch "recess for lid" plane through (20.5, 27.3, 8) normal (1, 0, 0) x (0, 1, 0) in component "case"
  line L0 (-28.8, -7.3) -> (-28.8, 9.5)
  line L1 (-28.8, 9.5) -> (-28.8, -7.3)
  line L2 (-28.8, -7.3) -> (-28.8, -9.5)
  line L3 (-28.8, -9.5) -> (-28.8, -7.3)
  line L4 (28.8, 9.5) -> (28.7975, 9.5)
  line L5 (28.7975, 9.5) -> (20.0025, 9.5)
  line L6 (20.0025, 9.5) -> (20, 9.5)
  line L7 (20, 9.5) -> (-20, 9.5)
  line L8 (-20, 9.5) -> (-20.0025, 9.5)
  line L9 (-20.0025, 9.5) -> (-28.7975, 9.5)
  line L10 (-28.7975, 9.5) -> (-28.8, 9.5)
  line L11 (-28.8, 9.5) -> (-28.7975, 9.5)
  line L12 (-28.7975, 9.5) -> (-20.0025, 9.5)
  line L13 (-20.0025, 9.5) -> (-20, 9.5)
  line L14 (-20, 9.5) -> (20, 9.5)
  line L15 (20, 9.5) -> (20.0025, 9.5)
  line L16 (20.0025, 9.5) -> (28.7975, 9.5)
  line L17 (28.7975, 9.5) -> (28.8, 9.5)
  line L18 (27.3, 9.5) -> (-27.3, 9.5)
  line L19 (-27.3, 9.5) -> (27.3, 9.5)
  line L20 (-28.2, 9.5) -> (-28.8, 6.5)
  dimension "d486" = 3
  dimension "d487" = 0.6
  constraint coincident L9 L20.start
  constraint coincident L0 L20.end
  measures "d486" vertical distance of L20.start L20.end
  measures "d487" horizontal distance of L20.start L20.end
extrude "Extrude38" cut sketch "recess for lid" along normal mid plane 8 bodies 1 in component "case"
component "case" placed x (1, 0, 0) y (0, 1, 0) z (0, 0, 1) at (0, 0, 0)
component "tray" placed x (1, 0, 0) y (0, 1, 0) z (0, 0, 1) at (0.1, 0.15, 10.15)
component "lid" placed x (1, 0, 0) y (0, 1, 0) z (0, 0, 1) at (0, 0, 17.5)
equation "d216 = d215"
equation "d227 = d226"
equation "d311 = 1 mm + d362"
equation "d368 = d369"
equation "d371 = d370"
equation "d375 = d330"
equation "d381 = d380"
named bodies: "case", "tray"
